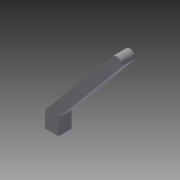
# Autodesk Inventor part: Funneling_v1
Saved by Autodesk Inventor 2013 (Build 170138000, 138)
## iProperties
Created: 2013-01-19
Part Number: Funneling_v1
Material: Generic
Document SubType Name: Modeling
Designer: motoennies
Density: 1 g/cm^3
Author: motoennies
Autodesk Inventor part; units mm, degrees
ref_plane "YZ Plane" through (0, 0, 0) normal (1, 0, 0) x (0, 1, 0)
ref_plane "XZ Plane" through (0, 0, 0) normal (0, 1, 0) x (-1, 0, 0)
ref_plane "XY Plane" through (0, 0, 0) normal (0, 0, 1) x (1, 0, 0)
sketch "Sketch1" plane through (0, 0, 0) normal (0, 0, 1) x (1, 0, 0)
  line L0 (0, 0) -> (0, 7.62)
  line L1 (0, 0) -> (6.35, 0)
  line L2 (6.35, 0) -> (6.35, 7.62)
  line L3 (0, 7.62) -> (31.9697, 45.72)
  line L4 (0, 7.62) -> (49.736, 7.62) construction
  line L5 (6.35, 7.62) -> (35.696, 42.5932)
  arc A0 (35.696, 42.5932) -> (31.9697, 45.72) centre (33.8329, 44.1566) ccw
  dimension "d0" = 7.62
  dimension "d1" = 6.35
  dimension "d2" = 50
  dimension "d3" = 38.1
  dimension "d4" = 45.6543
  dimension "d5" = 2.4322
  constraints: 12 end point, 2 perpendicular, 2 point on circle, 1 centre point, 1 equal length, 1 horizontal, 1 parallel, 1 tangent, 1 vertical
  measures "d0" distance of L0.start L0.end
  measures "d1" distance of L0.start L1.end
  measures "d2" angle of L4 L3
  measures "d3" vertical distance of L0.end L3.end
  measures "d4" distance of L2.end L5.end
  measures "d5" radius of A0
extrude "Extrusion1" add sketch "Sketch1" along normal blind 6.35
body "Solid1"
